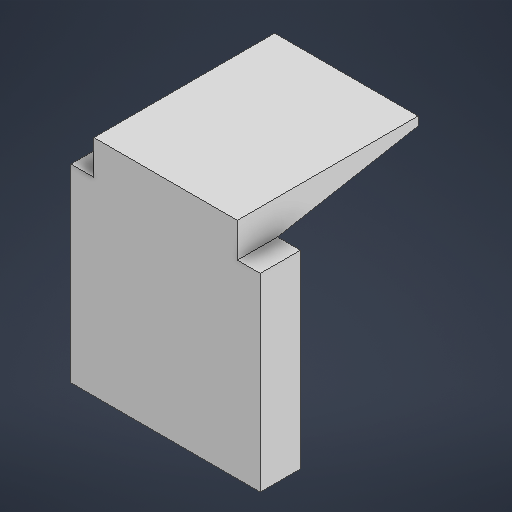
# Autodesk Inventor part: pan_base_holder_third
Saved by Autodesk Inventor 2026 (Build 300175000, 175)
## iProperties
Created: 2025-06-27
Part Number: pan_base_holder_third
Material: Generic
Document SubType Name: Modeling
Designer: user
Density: 1 g/cm^3
Appearance: Default
Author: user
Autodesk Inventor part; units mm, degrees
ref_plane "YZ Plane" through (0, 0, 0) normal (1, 0, 0) x (0, 1, 0)
ref_plane "XZ Plane" through (0, 0, 0) normal (0, 1, 0) x (-1, 0, 0)
ref_plane "XY Plane" through (0, 0, 0) normal (0, 0, 1) x (1, 0, 0)
sketch "Sketch1" plane through (0, 0, 0) normal (0, 0, 1) x (1, 0, 0)
  line L0 (-31, -31) -> (31, -31)
  line L1 (31, -31) -> (31, 31)
  line L2 (31, 31) -> (-31, 31)
  line L3 (-31, 31) -> (-31, -31)
  line L4 (-31, -31) -> (31, 31) construction
  line L5 (31, -31) -> (-31, 31) construction
  line L6 (-33, 33) -> (33, 33)
  line L7 (33, 33) -> (33, -33)
  line L8 (33, -33) -> (-33, -33)
  line L9 (-33, -33) -> (-33, 33)
  point P0 (0, 0)
  dimension "d0" = 62
  dimension "d1" = 62
  dimension "d2" = 2
  constraints: 20 end point, 4 parallel, 2 midpoint, 2 perpendicular, 1 horizontal, 3 other
  measures "d0" distance of L1.end L2.end
  measures "d1" distance of L0.end L1.end
  measures "d2" distance between parallel lines of L2 L6
extrude "Extrusion1" add sketch "Sketch1" along normal blind 2 contours L3 L2 L1 L0 | L6 L7 L8 L9
extrude "Extrusion2" add sketch "Sketch1" against normal blind 12
sketch "Sketch2" plane through (-33, 33, 2) normal (0, 1, 0) x (1, 0, 0)
  line L0 (8, 3) -> (58, 3)
  line L1 (58, 3) -> (58, 0)
  line L2 (58, 0) -> (8, 0)
  line L3 (8, 0) -> (8, 3)
  line L4 (0, 14) -> (0, 0) projected
  line L5 (0, 14) -> (66, 14) projected
  point P0 (33, 2)
  dimension "d7" = 50
  dimension "d8" = 3
  dimension "d9" = 8
  dimension "d10" = 11
  constraints: 8 end point, 2 parallel, 1 horizontal, 1 perpendicular
  measures "d7" distance of L1.end L2.end
  measures "d8" distance of L0.end L1.end
  measures "d9" distance between parallel lines of L4 L3
  measures "d10" distance between parallel lines of L5 L0
extrude "Extrusion3" add sketch "Sketch2" along normal blind 12
sketch "Sketch3" plane through (25, 33, -1) normal (0, 0, -1) x (-1, 0, 0)
  line L0 (50, 12) -> (0, 12) projected
  line L1 (50, 0) -> (50, 12) projected
  line L2 (0, 12) -> (50, 12)
  line L3 (50, 12) -> (50, 9)
  line L4 (50, 9) -> (0, 9)
  line L5 (0, 9) -> (0, 12)
  point P0 (25, -33)
  dimension "d13" = 3
  constraints: 8 end point, 2 parallel, 1 horizontal, 1 perpendicular, 1 point on line
  measures "d13" distance of L2.end L3.end
extrude "Extrusion4" add sketch "Sketch3" along normal blind 60
sketch "Sketch8" plane through (-25, 33, -1) normal (-1, 0, 0) x (0, 0, 1)
  line L0 (0, 9) -> (-60, 9) projected
  line L1 (0, 9) -> (-60, 9)
  line L2 (-60, 9) -> (-60, 0)
  line L3 (-60, 0) -> (0, 0)
  line L4 (0, 0) -> (0, 9)
  line L5 (-60, 9) -> (-10.9892, 0)
  point P0 (1, -33)
  dimension "d43" = 9
  constraints: 10 end point, 2 parallel, 1 horizontal, 1 perpendicular, 1 point on line
  measures "d43" distance of L2.end L1.end
extrude "Extrusion9" add sketch "Sketch8" against normal blind 2 contours L4 L3 L5 L0
ref_plane "Work Plane1" through (0, 33, 2) normal (1, 0, 0) x (0, 0, -1)
mirror "Mirror1" about plane through (0, 33, 2) normal (1, 0, 0) of "Extrusion9"
body "Solid1"
